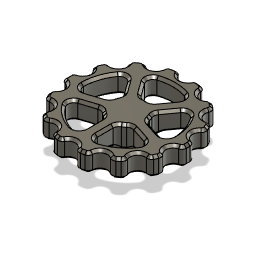
CR10_extruder_knob_ (Autodesk Fusion 360 design; units mm, degrees)
Autodesk Fusion 360 part; units mm, degrees
sketch "Sketch1" plane through (0, 0, 0) normal (0, 0, 1) x (1, 0, 0)
  line L0 (0, 0) -> (0, 10.5)
  line L1 (0, 10.5) -> (-20, 10.5)
  line L2 (-20, 10.5) -> (-20, 4.5)
  line L3 (-20, 4.5) -> (-5, 4.5)
  line L4 (-5, 4.5) -> (-5, 0)
  line L5 (-5, 0) -> (0, 0)
  dimension "d1" = 5
  dimension "d2" = 20
  dimension "d3" = 4.5
  dimension "d4" = 6
  constraint coincident L0.start L5.end
  constraint vertical L0
  constraint perpendicular L0 L1
  constraint perpendicular L1 L2
  constraint perpendicular L2 L3
  constraint perpendicular L3 L4
  constraint perpendicular L0 L5
  measures "d1" distance of L0 L4
  measures "d2" distance of L0.end L1.end
  measures "d3" distance of L3.end L4.end
  measures "d4" distance of L1.end L2.end
  measures "d12" diameter of L1.end
  measures "d28" distance of L1.end
revolve "Revolve1" add sketch "Sketch1" angle 360 about axis through (0, 0, 0) along (0, 1, 0)
sketch "Sketch2" plane through (0, 0, 0) normal (0, -1, 0) x (1, 0, 0)
  circle A0 centre (0, 0) radius 5
  circle A1 centre (0, 0) radius 2.625
  line L0 (-1.7847, 1.925) -> (1.7847, 1.925)
  line L1 (0, 1.925) -> (0, -2.625) construction
  dimension "d6" = 5.25
  dimension "d7" = 4.55
  constraint coincident A0.centre A1.centre
  constraint coincident A1 L0.start
  constraint horizontal L0
  constraint midpoint L0 L1.start
  constraint coincident A1 L1.end
  constraint perpendicular L0 L1
  measures "d6" diameter of A1
  measures "d7" distance of L0 L1.end
extrude "Extrude1" cut sketch "Sketch2" against normal blind 8 contours A1 L0 picked at (-0.5168, 0.5773)
chamfer "Chamfer1" distance 0.8 angle 45 2 edges at (0, 0, -2.625) (0, 0, 1.925)
fillet "Fillet1" radius 4 1 edges at (-4.6616, 4.5, 1.8081)
sketch "Sketch3" plane through (0, 10.5, 0) normal (0, 1, 0) x (-1, 0, 0)
  circle A0 centre (0, 0) radius 20
  circle A1 centre (0, 0) radius 20
  line L0 (0, 0) -> (0, -20.5)
  circle A2 centre (0, -20) radius 2.5
  dimension "d12" = 5
  constraint coincident A0.centre A1.centre
  constraint vertical L0
  constraint coincident L0 A2.centre
  constraint coincident A1 A2.centre
  measures "d12" diameter of A2
extrude "Extrude2" cut sketch "Sketch3" against normal blind 9 contours A0 A1 L0 A2 | A0 A1 A2 | A0 A1 L0 A2 picked at (-0.542, -20.7846)
fillet "Fillet2" radius 1.5 2 edges at (-2.4951, 7.5, -19.8438) (2.4951, 7.5, -19.8438)
pattern_circular "C-Pattern1" count 14 over 360 about axis through (0, 1.75, 0) along (0, 1, 0) of "Extrude2", "Fillet2"
chamfer "Chamfer2" distance 0.8 angle 45 56 edges at (18.0194, 10.5, 8.6777) (17.0584, 10.5, 9.8967) (13.6821, 10.5, 10.9111) (13.4445, 10.5, 14.4285) (12.4698, 10.5, 15.6366) (11.0751, 10.5, 16.318) (7.593, 10.5, 15.767) (5.8528, 10.5, 18.833) (4.4504, 10.5, 19.4986) (2.8982, 10.5, 19.5074) (0, 10.5, 17.5) (-2.8982, 10.5, 19.5074) (-4.4504, 10.5, 19.4986) (-5.8528, 10.5, 18.833) (-7.593, 10.5, 15.767) (-11.0751, 10.5, 16.318) (-12.4698, 10.5, 15.6366) (-13.4445, 10.5, 14.4285) (-13.6821, 10.5, 10.9111) (-17.0584, 10.5, 9.8967) (-18.0194, 10.5, 8.6777) (-18.3734, 10.5, 7.1663) (-17.0612, 10.5, 3.8941) (-19.6632, 10.5, 1.5153) (-20, 10.5, 0) (-19.6632, 10.5, -1.5153) (-17.0612, 10.5, -3.8941) (-18.3734, 10.5, -7.1663) (-18.0194, 10.5, -8.6777) (-17.0584, 10.5, -9.8967) (-13.6821, 10.5, -10.9111) (-13.4445, 10.5, -14.4285) (-12.4698, 10.5, -15.6366) (-11.0751, 10.5, -16.318) (-7.593, 10.5, -15.767) (-5.8528, 10.5, -18.833) (-4.4504, 10.5, -19.4986) (-2.8982, 10.5, -19.5074) (0, 10.5, -17.5) (2.8982, 10.5, -19.5074) (4.4504, 10.5, -19.4986) (5.8528, 10.5, -18.833) (7.593, 10.5, -15.767) (11.0751, 10.5, -16.318) (12.4698, 10.5, -15.6366) (13.4445, 10.5, -14.4285) (13.6821, 10.5, -10.9111) (17.0584, 10.5, -9.8967) (18.0194, 10.5, -8.6777) (18.3734, 10.5, -7.1663) (17.0612, 10.5, -3.8941) (19.6632, 10.5, -1.5153) (20, 10.5, 0) (19.6632, 10.5, 1.5153) (17.0612, 10.5, 3.8941) (18.3734, 10.5, 7.1663)
sketch "Sketch4" plane through (0, 0, 0) normal (0, -1, 0) x (1, 0, 0)
  circle A0 centre (0, 0) radius 5
  line L0 (-2.0748, 2.725) -> (2.0748, 2.725)
  arc A1 (-2.0748, 2.725) -> (2.0748, 2.725) centre (0, 0) ccw
  circle A2 centre (0, 0) radius 6
  circle A3 centre (0, 0) radius 14.8661
  line L1 (2, 22) -> (-2, 22)
  line L2 (-2, 22) -> (-2, 0.0011)
  line L3 (-2, 0.0011) -> (2, 0.0011)
  line L4 (2, 0.0011) -> (2, 22)
  line L5 (2, 22) -> (-2, 0.0011) construction
  line L6 (-2, 22) -> (2, 0.0011) construction
  line L7 (-21.5413, 4.8963) -> (-0.619, -1.9018)
  line L8 (-0.619, -1.9018) -> (0.617, 1.9024)
  line L9 (-20.3052, 8.7005) -> (-21.5413, 4.8963)
  line L10 (0.617, 1.9024) -> (-20.3052, 8.7005)
  line L11 (-11.3132, -18.9739) -> (1.6174, -1.1764)
  line L12 (1.6174, -1.1764) -> (-1.6187, 1.1747)
  line L13 (-14.5493, -16.6228) -> (-11.3132, -18.9739)
  line L14 (-1.6187, 1.1747) -> (-14.5493, -16.6228)
  line L15 (14.5493, -16.6228) -> (1.6187, 1.1747)
  line L16 (1.6187, 1.1747) -> (-1.6174, -1.1764)
  line L17 (11.3132, -18.9739) -> (14.5493, -16.6228)
  line L18 (-1.6174, -1.1764) -> (11.3132, -18.9739)
  line L19 (20.3052, 8.7005) -> (-0.617, 1.9024)
  line L20 (-0.617, 1.9024) -> (0.619, -1.9018)
  line L21 (21.5413, 4.8963) -> (20.3052, 8.7005)
  line L22 (0.619, -1.9018) -> (21.5413, 4.8963)
  point P0 (0, 11.0005)
  dimension "d19" = 12
  dimension "d21" = 360
  dimension "d28" = 4
  constraint concentric A0 A2
  constraint concentric A2 A3
  constraint perpendicular L1 L2
  constraint parallel L1 L3
  constraint parallel L2 L4
  constraint horizontal L1
  constraint coincident L5 P0
  constraint coincident L6 P0
  measures "d19" diameter of A2
  measures "d28" distance of L15.start L17.start
extrude "Extrude3" cut sketch "Sketch4" against normal blind 27 contours A2 A3 L4 L19 | A2 A3 L15 L22 | A2 A3 L2 L10 | A2 A3 L11 L18 | A2 A3 L7 L14
fillet "Fillet3" radius 2 20 edges at (10.2767, 7.5, -10.742) (4.943, 6.8229, -3.4009) (5.998, 6.8229, -0.154) (14.628, 7.5, 2.65) (13.3919, 7.5, 6.4542) (2, 7.5, 14.7309) (2, 6.8229, 5.6569) (4.762, 6.8229, 3.6502) (-2, 7.5, 14.7309) (-2, 6.8229, 5.6569) (-4.762, 6.8229, 3.6502) (-13.3919, 7.5, 6.4542) (-14.628, 7.5, 2.65) (-5.998, 6.8229, -0.154) (-4.943, 6.8229, -3.4009) (-10.2767, 7.5, -10.742) (-1.707, 6.8229, -5.7521) (-7.0406, 7.5, -13.0931) (7.0406, 7.5, -13.0931) (1.707, 6.8229, -5.7521)
chamfer "Chamfer3" distance 0.8 angle 45 40 edges at (12.2966, 10.5, 6.9669) (8.7381, 10.5, 12.0269) (2.826, 10.5, 13.8477) (2, 10.5, 9.5783) (2.2679, 10.5, 5.9282) (3.5267, 10.5, 4.8541) (4.9372, 10.5, 3.9889) (8.4915, 10.5, 4.862) (10.4258, 10.5, -9.5419) (14.1385, 10.5, -4.5939) (14.0432, 10.5, 1.5915) (9.7276, 10.5, 1.0578) (6.3389, 10.5, -0.325) (5.7063, 10.5, -1.8541) (5.3193, 10.5, -3.463) (7.248, 10.5, -6.5735) (1.6497, 10.5, -6.1291) (0, 10.5, -6) (-1.6497, 10.5, -6.1291) (-4.012, 10.5, -8.9246) (-5.8532, 10.5, -12.8641) (0, 10.5, -14.8661) (5.8532, 10.5, -12.8641) (4.012, 10.5, -8.9246) (-6.3389, 10.5, -0.325) (-9.7276, 10.5, 1.0578) (-14.0432, 10.5, 1.5915) (-14.1385, 10.5, -4.5939) (-10.4258, 10.5, -9.5419) (-7.248, 10.5, -6.5735) (-5.3193, 10.5, -3.463) (-5.7063, 10.5, -1.8541) (-2.2679, 10.5, 5.9282) (-2, 10.5, 9.5783) (-2.826, 10.5, 13.8477) (-8.7381, 10.5, 12.0269) (-12.2966, 10.5, 6.9669) (-8.4915, 10.5, 4.862) (-4.9372, 10.5, 3.9889) (-3.5267, 10.5, 4.8541)
chamfer "Chamfer4" distance 0.8 angle 45 50 edges at (14.0432, 4.5, 1.5915) (14.1385, 4.5, -4.5939) (10.4258, 4.5, -9.5419) (7.7908, 4.5, -7.3205) (6.2144, 4.3907, -5.1508) (5.3177, 3.4847, -3.4468) (5.7063, 3.1458, -1.8541) (6.3348, 3.4903, -0.3296) (8.0552, 4.3907, 0.5144) (10.6058, 4.5, 1.3431) (2.826, 4.5, 13.8477) (8.7381, 4.5, 12.0269) (12.2966, 4.5, 6.9669) (9.3697, 4.5, 5.1473) (6.8191, 4.3907, 4.3186) (4.9254, 3.4871, 3.9914) (3.5267, 3.1458, 4.8541) (2.2711, 3.4903, 5.9228) (2, 4.3907, 7.8199) (2, 4.5, 10.5017) (-6.326, 3.4829, -0.3395) (-5.7063, 3.1458, -1.8541) (-5.318, 3.4867, -3.4503) (-6.2144, 4.3907, -5.1508) (-7.7908, 4.5, -7.3205) (-10.4258, 4.5, -9.5419) (-14.1385, 4.5, -4.5939) (-14.0432, 4.5, 1.5915) (-10.6058, 4.5, 1.3431) (-8.0552, 4.3907, 0.5144) (-12.2966, 4.5, 6.9669) (-8.7381, 4.5, 12.0269) (-2.826, 4.5, 13.8477) (-2, 4.5, 10.5017) (-2, 4.3907, 7.8199) (-2.278, 3.4826, 5.911) (-3.5267, 3.1458, 4.8541) (-4.9277, 3.4883, 3.9909) (-6.8191, 4.3907, 4.3186) (-9.3697, 4.5, 5.1473) (-1.6343, 3.4843, -6.1223) (0, 3.1458, -6) (1.6384, 3.4869, -6.1241) (2.9784, 4.3907, -7.502) (4.5547, 4.5, -9.6716) (5.8532, 4.5, -12.8641) (0, 4.5, -14.8661) (-5.8532, 4.5, -12.8641) (-4.5547, 4.5, -9.6716) (-2.9784, 4.3907, -7.502)
chamfer "Chamfer5" distance 0.8 angle 45 56 edges at (-12.4698, 4.5, -15.6366) (-13.4445, 4.5, -14.4285) (-13.6821, 4.5, -10.9111) (-17.0584, 4.5, -9.8967) (-18.0194, 4.5, -8.6777) (-18.3734, 4.5, -7.1663) (-17.0612, 4.5, -3.8941) (-19.6632, 4.5, -1.5153) (-20, 4.5, 0) (-19.6632, 4.5, 1.5153) (-17.0612, 4.5, 3.8941) (-18.3734, 4.5, 7.1663) (-18.0194, 4.5, 8.6777) (-17.0584, 4.5, 9.8967) (-13.6821, 4.5, 10.9111) (-13.4445, 4.5, 14.4285) (-12.4698, 4.5, 15.6366) (-11.0751, 4.5, 16.318) (-7.593, 4.5, 15.767) (-5.8528, 4.5, 18.833) (-4.4504, 4.5, 19.4986) (-2.8982, 4.5, 19.5074) (0, 4.5, 17.5) (2.8982, 4.5, 19.5074) (4.4504, 4.5, 19.4986) (5.8528, 4.5, 18.833) (7.593, 4.5, 15.767) (11.0751, 4.5, 16.318) (12.4698, 4.5, 15.6366) (13.4445, 4.5, 14.4285) (13.6821, 4.5, 10.9111) (17.0584, 4.5, 9.8967) (18.0194, 4.5, 8.6777) (18.3734, 4.5, 7.1663) (17.0612, 4.5, 3.8941) (19.6632, 4.5, 1.5153) (20, 4.5, 0) (19.6632, 4.5, -1.5153) (17.0612, 4.5, -3.8941) (18.3734, 4.5, -7.1663) (18.0194, 4.5, -8.6777) (17.0584, 4.5, -9.8967) (13.6821, 4.5, -10.9111) (13.4445, 4.5, -14.4285) (12.4698, 4.5, -15.6366) (11.0751, 4.5, -16.318) (7.593, 4.5, -15.767) (5.8528, 4.5, -18.833) (4.4504, 4.5, -19.4986) (2.8982, 4.5, -19.5074) (0, 4.5, -17.5) (-2.8982, 4.5, -19.5074) (-4.4504, 4.5, -19.4986) (-5.8528, 4.5, -18.833) (-7.593, 4.5, -15.767) (-11.0751, 4.5, -16.318)
